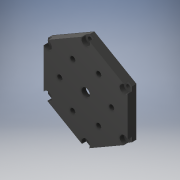
# Autodesk Inventor part: TA01
Saved by Autodesk Inventor 2017 (Build 210142000, 142)
## iProperties
Created: 2018-10-09
Part Number: TA01
Material: ABS Plastic
Document SubType Name: Modeling
Designer: Zach
Density: 1.06 g/cm^3
Appearance: Smooth - Black
Author: Zach
Autodesk Inventor part; units mm, degrees
ref_plane "YZ Plane" through (0, 0, 0) normal (1, 0, 0) x (0, 1, 0)
ref_plane "XZ Plane" through (0, 0, 0) normal (0, 1, 0) x (-1, 0, 0)
ref_plane "XY Plane" through (0, 0, 0) normal (0, 0, 1) x (1, 0, 0)
sketch "Sketch1" plane through (0, 0, 0) normal (0, 0, 1) x (1, 0, 0)
  circle A0 centre (0, 0) radius 5
  circle A1 centre (-30, 0) radius 3
  circle A2 centre (-15, -25.9808) radius 3
  circle A3 centre (15, -25.9808) radius 3
  circle A4 centre (30, 0) radius 3
  circle A5 centre (15, 25.9808) radius 3
  circle A6 centre (-15, 25.9808) radius 3
  line L0 (0, 56) -> (48.4974, 28)
  line L1 (48.4974, 28) -> (48.4974, -28)
  line L2 (48.4974, -28) -> (0, -56)
  line L3 (0, -56) -> (-48.4974, -28)
  line L4 (-48.4974, -28) -> (-48.4974, 28)
  line L5 (-48.4974, 28) -> (0, 56)
  point P0 (48.4974, 0)
  dimension "d0" = 10
  dimension "d2" = 6
  dimension "d6" = 360
  dimension "d15" = 30
  dimension "d33" = 112
  constraints: 12 end point, 7 centre point, 2 coincident, 2 horizontal alignment, 1 midpoint, 26 other
  measures "d0" diameter of A0
  measures "d2" diameter of A1
  measures "d15" distance of point (0, 0) A1.centre
  measures "d33" distance of L2.end L0.start
extrude "Extrusion1" add sketch "Sketch1" along normal blind 10
sketch "Sketch7" plane through (0, 0, 10) normal (0, 0, 1) x (1, 0, 0)
  circle A0 centre (0, 51) radius 2.5
  line L0 (48.4974, 28) -> (0, 56) projected
  circle A1 centre (-44.1673, 25.5) radius 2.5
  circle A2 centre (-44.1673, -25.5) radius 2.5
  circle A3 centre (0, -51) radius 2.5
  circle A4 centre (44.1673, -25.5) radius 2.5
  circle A5 centre (44.1673, 25.5) radius 2.5
  point P0 (0, 0)
  dimension "d42" = 5
  dimension "d43" = 5
  dimension "d46" = 360
  constraints: 6 centre point, 1 vertical alignment, 13 other
  measures "d42" diameter of A0
  measures "d43" distance of L0.end A0.centre
extrude "Extrusion6" cut sketch "Sketch7" against normal through all
sketch "Sketch8" plane through (0, 0, 10) normal (0, 0, 1) x (1, 0, 0)
  circle A0 centre (0, 51) radius 2.5 projected
  line L0 (0, 56) -> (-48.4974, 28) projected
  circle A1 centre (0, 51) radius 5
  circle A2 centre (-44.1673, 25.5) radius 5
  circle A3 centre (-44.1673, -25.5) radius 5
  circle A4 centre (0, -51) radius 5
  circle A5 centre (44.1673, -25.5) radius 5
  circle A6 centre (44.1673, 25.5) radius 5
  point P0 (0, 0)
  point P1 (-48.4974, 28)
  point P2 (-48.4974, -28)
  point P3 (0, -56)
  point P4 (48.4974, -28)
  point P5 (48.4974, 28)
  dimension "d52" = 360
  constraints: 2 vertical alignment, 1 coincident, 35 other
extrude "Extrusion7" cut sketch "Sketch8" against normal blind 5 contours A0 | A1 L0 | L0 A1 | A2 L0 | L0 A2 | A3 | A4 | A5 | A6
sketch "Sketch9" plane through (0, 0, 0) normal (0, 0, -1) x (-1, 0, 0)
  circle A0 centre (0, 0) radius 25
  dimension "d56" = 50
  constraints: 1 centre point, 1 coincident
  measures "d56" diameter of A0
extrude "Extrusion8" cut sketch "Sketch9" against normal blind 5
body "Solid1"
